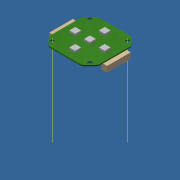
# Autodesk Inventor part: encoder_neu
Saved by Autodesk Inventor 2016 (Build 200138000, 138)
## iProperties
Created: 2015-01-07
Part Number: encoder_neu
Material: Generisch
Document SubType Name: Modeling
Designer: 4ndreas
Density: 1 g/cm^3
Appearance: PCB- green
Mass: 2.89597 g
Surface Area: 48.7766 cm^2
Volume: 2.89597 cm^3
Description: Encoder with LEDs
Author: 4ndreas
Autodesk Inventor part; units mm, degrees
ref_plane "YZ Plane" through (0, 0, 0) normal (1, 0, 0) x (0, 1, 0)
ref_plane "XZ Plane" through (0, 0, 0) normal (0, 1, 0) x (-1, 0, 0)
ref_plane "XY Plane" through (0, 0, 0) normal (0, 0, 1) x (1, 0, 0)
sketch "Skizze1" plane through (0, 0, 0) normal (0, 0, 1) x (1, 0, 0)
  circle A0 centre (0, 0) radius 25
  circle A1 centre (0, 0) radius 22.6274 construction
  line L0 (-16, 16) -> (16, 16) construction
  line L1 (16, 16) -> (16, -16) construction
  line L2 (16, -16) -> (-16, -16) construction
  line L3 (-16, -16) -> (-16, 16) construction
  line L4 (-21, -21) -> (21, -21)
  line L5 (21, -21) -> (21, 21)
  line L6 (21, 21) -> (-21, 21)
  line L7 (-21, 21) -> (-21, -21)
  line L8 (-21, -21) -> (21, 21) construction
  line L9 (21, -21) -> (-21, 21) construction
  point P0 (16, 16)
  dimension "d2" = 32
  dimension "d92" = 50
  dimension "d95" = 42
  constraints: 20 end point, 5 coincident, 4 parallel, 4 perpendicular, 4 point on circle, 2 centre point, 2 horizontal, 2 midpoint, 1 point on line
  measures "d2" distance between parallel lines of L1 L3
  measures "d92" diameter of A0
  measures "d95" distance between parallel lines of L5 L7
extrude "Extrusion1" add sketch "Skizze1" against normal blind 1 contours A0 L5 | L5 A0 L4 L7 L6 | L6 A0 | A0 L4 | L7 A0
hole "Bohrung1" at (-16, 16, 0) at (16, 16, 0) at (16, -16, 0) at (-16, -16, 0) direction (0, 0, -1) diameter 3.2 end through all
sketch "Skizze2" plane through (0, 0, 0) normal (0, 0, 1) x (1, 0, 0)
  circle A0 centre (16, -16) radius 1.6 projected
  circle A1 centre (-16, 16) radius 1.6 projected
  circle A2 centre (16, 16) radius 1.6 projected
  circle A3 centre (-16, -16) radius 1.6 projected
  circle A4 centre (0, 0) radius 25 projected
  line L0 (-25.6213, 25.3721) -> (25.184, 25.3721) construction
  line L1 (25.184, 25.3721) -> (25.184, -25.4332) construction
  line L2 (25.184, -25.4332) -> (-25.6213, -25.4332) construction
  line L3 (-25.6213, -25.4332) -> (-25.6213, 25.3721) construction
  constraints: 1 horizontal, 2 other
sketch "Skizze3" plane through (0, 0, 0) normal (0, 0, 1) x (1, 0, 0)
  circle A0 centre (0, 0) radius 25 projected
  line L0 (-2.5, 2.5) -> (2.5, 2.5)
  line L1 (2.5, 2.5) -> (2.5, -2.5)
  line L2 (2.5, -2.5) -> (-2.5, -2.5)
  line L3 (-2.5, -2.5) -> (-2.5, 2.5)
  line L4 (-15, 2.5) -> (-10, 2.5)
  line L5 (-10, 2.5) -> (-10, -2.5)
  line L6 (-10, -2.5) -> (-15, -2.5)
  line L7 (-15, -2.5) -> (-15, 2.5)
  line L8 (-15, 2.5) -> (-10, -2.5) construction
  line L9 (-2.5, 2.5) -> (2.5, -2.5) construction
  line L10 (2.5, -2.5) -> (0, 0) construction
  line L11 (0, 0) -> (-12.5, 0) construction
  line L12 (-2.5, -15) -> (-2.5, -10)
  line L13 (-2.5, -10) -> (2.5, -10)
  line L14 (2.5, -10) -> (2.5, -15)
  line L15 (2.5, -15) -> (-2.5, -15)
  line L16 (15, -2.5) -> (10, -2.5)
  line L17 (10, -2.5) -> (10, 2.5)
  line L18 (10, 2.5) -> (15, 2.5)
  line L19 (15, 2.5) -> (15, -2.5)
  line L20 (2.5, 15) -> (2.5, 10)
  line L21 (2.5, 10) -> (-2.5, 10)
  line L22 (-2.5, 10) -> (-2.5, 15)
  line L23 (-2.5, 15) -> (2.5, 15)
  dimension "d24" = 5
  dimension "d25" = 12.5
  dimension "d28" = 360
  constraints: 49 end point, 5 parallel, 3 equal length, 3 horizontal, 2 midpoint, 2 perpendicular, 1 collinear, 33 other
  measures "d24" distance between parallel lines of L1 L3
  measures "d25" distance of L10.end L11.end
extrude "Extrusion2" add sketch "Skizze3" along normal blind 1.6 separate body contours L0 L1 L2 L3 | L4 L5 L6 L7 | L12 L13 L14 L15 | L16 L17 L18 L19 | L20 L21 L22 L23
sketch "Skizze4" plane through (0, 0, -1) normal (0, 0, -1) x (-1, 0, 0)
  circle A0 centre (0, 0) radius 25 projected
  line L0 (-2.95, 2.5) -> (2.95, 2.5)
  line L1 (2.95, 2.5) -> (2.95, -2.5)
  line L2 (2.95, -2.5) -> (-2.95, -2.5)
  line L3 (-2.95, -2.5) -> (-2.95, 2.5)
  line L4 (-2.95, -2.5) -> (2.95, 2.5) construction
  dimension "d33" = 5.9
  dimension "d34" = 5
  constraints: 10 end point, 2 parallel, 1 coincident, 1 horizontal, 1 midpoint, 1 perpendicular
  measures "d33" distance between parallel lines of L3 L1
  measures "d34" distance between parallel lines of L2 L0
extrude "Extrusion3" add sketch "Skizze4" along normal blind 2 separate body contours L0 L1 L2 L3
sketch "Skizze5" plane through (0, 0, -1) normal (0, 0, -1) x (-1, 0, 0)
  circle A0 centre (0, 0) radius 25 projected
  line L0 (-24.5, 10) -> (-19.5, 10)
  line L1 (-19.5, 10) -> (-19.5, -10)
  line L2 (-19.5, -10) -> (-24.5, -10)
  line L3 (-24.5, -10) -> (-24.5, 10)
  line L4 (19.5, 10) -> (24.5, 10)
  line L5 (24.5, 10) -> (24.5, -10)
  line L6 (24.5, -10) -> (19.5, -10)
  line L7 (19.5, -10) -> (19.5, 10)
  line L8 (-24.5, 0) -> (24.5, 0) construction
  line L9 (-22, 10) -> (-22, -10) construction
  point P0 (0, 0)
  dimension "d38" = 20
  dimension "d39" = 5
  dimension "d40" = 22
  constraints: 20 end point, 5 midpoint, 4 parallel, 3 perpendicular, 2 equal length, 2 horizontal, 1 coincident
  measures "d38" distance between parallel lines of L2 L0
  measures "d39" distance between parallel lines of L3 L1
  measures "d40" distance from line of L9 A0.centre
extrude "Extrusion4" add sketch "Skizze5" along normal blind 5 contours L5 A0 L6 L7 L4 | A0 L4 L5 | L5 L6 A0 | L0 L1 L2 A0 L3 | A0 L3 L0 | L2 L3 A0 bodies 3
sketch "Skizze6" plane through (0, 0, -1) normal (0, 0, -1) x (-1, 0, 0)
  line L0 (-26.2075, 26.1914) -> (26.4628, 26.1914) construction
  line L1 (26.4628, 26.1914) -> (26.4628, -26.479) construction
  line L2 (26.4628, -26.479) -> (-26.2075, -26.479) construction
  line L3 (-26.2075, -26.479) -> (-26.2075, 26.1914) construction
  constraints: 1 horizontal, 2 other
sketch "Skizze7" plane through (0, 0, 0) normal (0, 0, 1) x (1, 0, 0)
  line L0 (-21, -21) -> (21, -21)
  line L1 (21, -21) -> (21, 21)
  line L2 (21, 21) -> (-21, 21)
  line L3 (-21, 21) -> (-21, -21)
  line L4 (-21, -21) -> (21, 21) construction
  line L5 (21, -21) -> (-21, 21) construction
  line L6 (-26, -26) -> (26, -26)
  line L7 (26, -26) -> (26, 26)
  line L8 (26, 26) -> (-26, 26)
  line L9 (-26, 26) -> (-26, -26)
  line L10 (-26, -26) -> (26, 26) construction
  line L11 (26, -26) -> (-26, 26) construction
  point P0 (0, 0)
  dimension "d96" = 42
  dimension "d97" = 52
  constraints: 24 end point, 4 midpoint, 4 parallel, 3 perpendicular, 2 horizontal, 1 collinear
  measures "d96" distance between parallel lines of L1 L3
  measures "d97" distance between parallel lines of L7 L9
extrude "Extrusion5" cut sketch "Skizze7" against normal through all bodies 1
